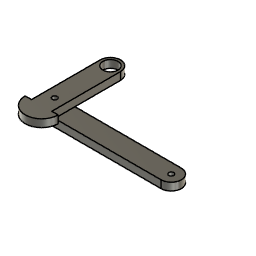
Servo Parallel Linkage v3 (Autodesk Fusion 360 design; units mm, degrees)
Autodesk Fusion 360 part; units mm, degrees
sketch "Sketch1" plane through (0, 0, 0) normal (0, 0, 1) x (1, 0, 0)
  line L0 (-11.5, 2) -> (11.5, 2)
  line L1 (11.5, -2) -> (-11.5, -2)
  line L2 (-13.5, 2) -> (13.5, -2) construction
  line L3 (13.5, 2) -> (-13.5, -2) construction
  arc A0 (-11.5, 2) -> (-13.5, 0) centre (-11.5, 0) ccw
  arc A1 (-13.5, 0) -> (-11.5, -2) centre (-11.5, 0) ccw
  arc A2 (13.5, 0) -> (11.5, 2) centre (11.5, 0) ccw
  arc A3 (11.5, -2) -> (13.5, 0) centre (11.5, 0) ccw
  circle A4 centre (-11.5, 0) radius 0.5
  circle A5 centre (11.5, 0) radius 0.5
  dimension "d1" = 27
  dimension "d2" = 4
  dimension "d3" = 2
  dimension "d4" = 2
  dimension "d5" = 1
  dimension "d6" = 1
  constraint horizontal L0
  constraint parallel L0 L1
  constraint coincident L2 origin
  constraint coincident L3 origin
  constraint coincident L2.start L0
  constraint tangent L0 A0
  constraint coincident L3.end L1
  constraint tangent L1 A1
  constraint coincident A0.end A1.start
  constraint coincident L3.start L0
  constraint tangent L0 A2
  constraint equal A1 A2
  constraint coincident L2.end L1
  constraint tangent L1 A3
  constraint equal A1 A3
  constraint coincident A2.start A3.end
  constraint concentric A0 A4
  constraint concentric A2 A5
  measures "d1" distance of L2.end L3.end
  measures "d2" distance of L3.start L2.end
  measures "d3" radius of A0
  measures "d4" radius of A1
  measures "d5" diameter of A4
  measures "d6" diameter of A5
extrude "Extrude1" add sketch "Sketch1" along normal blind 1.5
sketch "Sketch2" plane through (0, 0, 1.5) normal (0, 0, 1) x (-1, 0, 0)
  circle A0 centre (-11.5, 0) radius 0.5
  circle A1 centre (11.5, 0) radius 0.5
  arc A2 (11.5, -2) -> (11.5, 2) centre (11.5, 0) ccw
  line L0 (11.5, 2) -> (-11.5, 2)
  arc A3 (-11.5, 2) -> (-11.5, -2) centre (-11.5, 0) ccw
  line L1 (-11.5, -2) -> (11.5, -2)
  line L2 (9.5, 0) -> (9.5, -11)
  line L3 (13.5, -11) -> (13.5, 0)
  line L4 (13.5, 0) -> (13.5, 2.5617)
  line L5 (9.5, 2.5617) -> (9.5, 0)
  line L6 (9.5, 2.5617) -> (9.5, 2.5)
  line L7 (8.0446, 2.5617) -> (8.7247, 2.5617)
  arc A4 (14.75, 2.5617) -> (8.25, 2.5617) centre (11.5, 2.5617) ccw
  line L8 (14.75, 2.5617) -> (13.5, 2.5617)
  line L9 (9.5, 2.5617) -> (8.25, 2.5617)
  arc A5 (9.5, -11) -> (11.5, -13) centre (11.5, -11) ccw
  arc A6 (11.5, -13) -> (13.5, -11) centre (11.5, -11) ccw
  circle A7 centre (11.5, -11) radius 1.5
  point P0 (13.5, -13)
  dimension "d9" = 4
  dimension "d10" = 13
  dimension "d12" = 6.5
  dimension "d13" = 2
  dimension "d14" = 2
  dimension "d15" = 3
  constraint vertical L2
  constraint vertical L3
  constraint midpoint A2 L3.end
  constraint vertical L4
  constraint vertical L5
  constraint perpendicular L6 L8
  constraint coincident L7.end L8
  constraint coincident L5.start L8
  constraint coincident L5 L6.end
  constraint collinear L8 L9
  constraint tangent L2 A5
  constraint coincident P0 L3
  constraint tangent L3 A6
  constraint coincident A5.end A6.start
  constraint concentric A6 A7
  measures "d9" distance of L3.end L2.start
  measures "d10" distance of L3.end P0
  measures "d12" diameter of A4
  measures "d13" radius of A5
  measures "d14" radius of A6
  measures "d15" diameter of A7
extrude "Extrude2" add sketch "Sketch2" along normal blind 1.5 contours A2 L0 L1 L2 L5 | A2 L1 L2 L3 A5 A6 | A2 L0 L4 L5 L6 L7 A4 L8 L9
equation "d9 = 1 mm + 1.5 mm + 1.5 mm"
equation "d10 = 10.5 mm + 2.5 mm"
named bodies: "Top Part"
